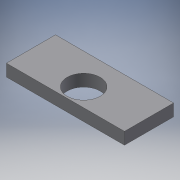
# Autodesk Inventor part: CHAPA_APOIO_CASTANHA_EIXO_Z
Saved by Autodesk Inventor 2018 (Build 220112000, 112)
## iProperties
Created: 2018-10-11
Part Number: CHAPA_APOIO_CASTANHA_EIXO_Z
Material: Genérico
Document SubType Name: Modeling
Designer: Usuario
Density: 1 g/cm^3
Appearance: Padrão
Author: Usuario
Autodesk Inventor part; units mm, degrees
ref_plane "YZ Plane" through (0, 0, 0) normal (1, 0, 0) x (0, 1, 0)
ref_plane "XZ Plane" through (0, 0, 0) normal (0, 1, 0) x (-1, 0, 0)
ref_plane "XY Plane" through (0, 0, 0) normal (0, 0, 1) x (1, 0, 0)
sketch "Esboço1" plane through (0, 0, 0) normal (0, 0, 1) x (1, 0, 0)
  line L0 (0, 12.7) -> (125, 12.7)
  line L1 (125, 12.7) -> (125, -39.3)
  line L2 (125, -39.3) -> (0, -39.3)
  line L3 (0, -39.3) -> (0, 12.7)
  circle A0 centre (62.5, -20) radius 11.5
  dimension "d0" = 52
  dimension "d1" = 23
  dimension "d2" = 125
  constraints: 8 end point, 2 parallel, 1 centre point, 1 horizontal, 1 perpendicular
  measures "d0" distance of L0.end L1.end
  measures "d1" diameter of A0
  measures "d2" distance of L1.end L2.end
extrude "Extrusão1" add sketch "Esboço1" along normal blind 12.7
sketch "Esboço2" plane through (0, 0, 12.7) normal (0, 0, 1) x (1, 0, 0)
  circle A0 centre (46.5, -20) radius 1 construction
  circle A1 centre (51.1863, -31.3137) radius 1 construction
  circle A2 centre (51.1863, -8.6863) radius 1 construction
  circle A3 centre (73.8137, -8.6863) radius 1 construction
  circle A4 centre (78.5, -20) radius 1 construction
  circle A5 centre (73.8137, -31.3137) radius 1 construction
  point P0 (0, 0)
  dimension "d5" = 2
  dimension "d6" = 2
  dimension "d7" = 2
  dimension "d8" = 2
  dimension "d9" = 2
  dimension "d10" = 2
  constraints: 6 centre point
  measures "d5" diameter of A0
  measures "d6" diameter of A1
  measures "d7" diameter of A2
  measures "d8" diameter of A3
  measures "d9" diameter of A4
  measures "d10" diameter of A5
hole "Furo1" at (46.5, -20, 12.7) at (51.1863, -31.3137, 12.7) at (51.1863, -8.6863, 12.7) at (73.8137, -8.6863, 12.7) at (78.5, -20, 12.7) at (73.8137, -31.3137, 12.7) direction (0, 0, -1) diameter 4.134 end through all thread size "M5x0.8" class "6H" standard "ANSI Metric M Profile"
